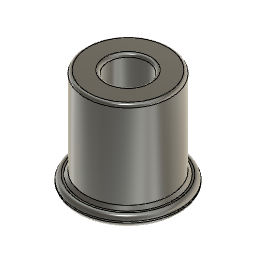
cafelat_tamper_sleeve_v1 (Autodesk Fusion 360 design; units mm, degrees)
Autodesk Fusion 360 part; units mm, degrees
note: some values were not read from the file. Set by a fixed rule: which face or edge a step refers to.
sketch "Sketch2" plane through (0, 0, 0) normal (0, 0, 1) x (1, 0, 0)
  circle A0 centre (0, 0) radius 28.75
  circle A1 centre (0, 0) radius 13.2
  dimension "d1" = 57.5
  dimension "d2" = 26.4
  constraint coincident A0.centre A1.centre
  measures "d1" diameter of A0
  measures "d2" diameter of A1
sketch "Sketch3" plane through (0, 0, 80) normal (0, 0, 1) x (-1, 0, 0)
  circle A0 centre (0, 0) radius 13.2
  circle A1 centre (0, 0) radius 28.75
  circle A2 centre (0, 0) radius 31.75
  dimension "d5" = 63.5
  constraint coincident A0.centre A1.centre
  measures "d5" diameter of A2
sketch "Sketch4" plane through (0, 0, 0) normal (0, 0, 1) x (1, 0, 0)
  circle A0 centre (0, 0) radius 28.95
  circle A1 centre (0, 0) radius 13.225
  dimension "d11" = 57.9
  dimension "d12" = 26.45
  constraint coincident A0.centre A1.centre
  constraint concentric A0 A1
  measures "d11" diameter of A0
  measures "d12" diameter of A1
extrude "Extrude3" add sketch "Sketch4" along normal blind 59.1 makes body 1
sketch "Sketch5" plane through (0, 0, 0) normal (0, 0, 1) x (1, 0, 0)
  circle A0 centre (0, 0) radius 10.285
  dimension "d15" = 20.57
  constraint coincident A0.centre origin
  measures "d15" diameter of A0
extrude "Extrude4" add sketch "Sketch5" along normal blind 7.35 separate body makes body 2
fillet "Fillet4" radius 4 1 edges at (-12.33, 4.7824, 59.1) on bodies 1
chamfer "Chamfer1" distance 0.5 angle 45 1 edges at (-26.9909, -10.4688, 59.1) on bodies 1
fillet "Fillet5" radius 2 1 edges at (-9.589, -3.7192, 7.35) on bodies 2
sketch "Sketch6" plane through (0, 0, 0) normal (0, 0, 1) x (1, 0, 0)
  circle A0 centre (0, 0) radius 35
  dimension "d21" = 70
  constraint coincident A0.centre origin
  measures "d21" diameter of A0
extrude "Extrude5" add sketch "Sketch6" against normal blind 20 bodies 1 2
fillet "Fillet6" radius 15 1 edges at (-32.6315, 12.6565, -20) on bodies 1
move_face "OffsetFaces1" offset -0.5 1 faces at (13.2086, -0.6592, 36.7333) on bodies 1
delete_face "DeleteFace1" 1 faces at (-10.1244, -1.0131, 6.0041) on bodies 1
move_face "OffsetFaces2" offset -0.1 1 faces at (10.2722, 0.5127, 2.45) on bodies 1
delete_face "DeleteFace2" 1 faces at (27.8933, -7.1025, 58.7667) on bodies 1
delete_face "DeleteFace3" 1 faces at (3.0476, 17.2839, 59.0962) on bodies 1
move_face "OffsetFaces3" offset 2 1 faces at (23.7672, 1.4383, 59.1) on bodies 1
chamfer "Chamfer2" distance 2 angle 45 1 edges at (-26.9909, 10.4688, 61.1) on bodies 1
fillet "Fillet7" radius 5 1 edges at (-12.7962, 4.9632, 61.1) on bodies 1
fillet "Fillet8" radius 1 1 edges at (-32.6315, -12.6565, 0) on bodies 1
fillet "Fillet9" radius 2 1 edges at (-9.4958, 3.6831, 7.35) on bodies 1
delete_face "DeleteFace4" 1 faces at (16.2532, 8.851, 61.0952) on bodies 1
delete_face "DeleteFace5" 1 faces at (10.0249, 1.0031, 6.0041) on bodies 1
delete_face "DeleteFace6" 1 faces at (-7.6603, 27.2262, 59.7667) on bodies 1
move_face "OffsetFaces4" offset -0.2 1 faces at (-28.8061, 2.8825, 40.7333) on bodies 1
move_face "OffsetFaces5" offset 0.325 1 faces at (13.7079, 0.6841, 20.3667) on bodies 1
move_face "OffsetFaces6" offset 0.115 1 faces at (10.1723, 0.5077, 2.45) on bodies 1
sketch "Sketch7" plane through (0, 0, 0) normal (0, 1, 0) x (1, 0, 0)
move_face "OffsetFaces7" offset 3 1 faces at (3.3442, 1.8576, 7.35) on bodies 1
fillet "Fillet10" radius 2 1 edges at (-9.603, -3.7246, 10.35) on bodies 1
fillet "Fillet11" radius 2 1 edges at (-12.4932, -4.8456, 61.1) on bodies 1
fillet "Fillet12" radius 2 1 edges at (-26.8044, -10.3964, 61.1) on bodies 1
delete_face "DeleteFace7" 1 faces at (-34.7289, 1.7332, -7.6047) on bodies 1
fillet "Fillet13" radius 5 1 edges at (-32.6315, -12.6565, -20) on bodies 1
delete_face "DeleteFace8" 1 faces at (-34.7254, 1.7331, -16.5035) on bodies 1
move_face "OffsetFaces8" offset -10 1 faces at (2.1399, 9.8952, -20) on bodies 1
fillet "Fillet14" radius 5 1 edges at (-32.6315, 12.6565, -10) on bodies 1
delete_face "DeleteFace9" 1 faces at (-34.7254, -1.7331, -6.5035) on bodies 1
move_face "OffsetFaces9" offset -3 1 faces at (2.1399, 9.8952, -10) on bodies 1
fillet "Fillet15" radius 3 1 edges at (-32.6315, -12.6565, -7) on bodies 1
delete_face "DeleteFace10" 1 faces at (14.3923, 31.8965, -0.8839) on bodies 1
fillet "Fillet16" radius 3 1 edges at (-32.6315, 12.6565, 0) on bodies 1
chamfer "Chamfer3" distance 2 angle 45 1 edges at (-26.8044, -10.3964, 0) on bodies 1
